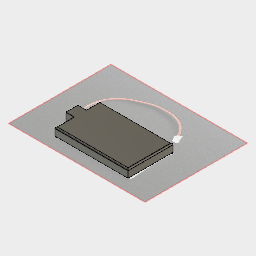
LiPo Battery (Autodesk Fusion 360 design; units mm, degrees)
Autodesk Fusion 360 part; units mm, degrees
sketch "Sketch1" plane through (0, 0, 0) normal (0, 0, 1) x (1, 0, 0) in component "LiPo_Battery"
  line L0 (33, 4) -> (-27, 4)
  line L1 (-27, -33) -> (33, -33)
  line L2 (33, -33) -> (33, 4)
  line L3 (-27, -8) -> (-33, -8)
  line L4 (-33, -8) -> (-33, -18)
  line L5 (-33, -18) -> (-27, -18)
  line L6 (-27, 4) -> (-27, -8)
  line L7 (-27, -18) -> (-27, -33)
  dimension "d4" = 60
  dimension "d5" = 37
  dimension "d6" = 6
  dimension "d7" = 10
  constraint horizontal L0
  constraint vertical L6
  constraint horizontal L1
  constraint vertical L2
  constraint horizontal L3
  constraint vertical L4
  constraint horizontal L5
  constraint collinear L6 L7
  measures "d5" distance of L0 L1
extrude "Extrude1" add sketch "Sketch1" along normal blind 7.5 in component "LiPo_Battery"
fillet "Fillet1" radius 1 10 edges at (3, -33, 7.5) (-27, -2, 7.5) (-27, -25.5, 7.5) (3, 4, 7.5) (33, -14.5, 7.5) (3, -33, 0) (33, -14.5, 0) (3, 4, 0) (-27, -25.5, 0) (-27, -2, 0) in component "LiPo_Battery"
sketch "Sketch2" plane through (0, 0, 7.5) normal (0, 0, 1) x (-1, 0, 0) in component "LiPo_Battery"
  line L0 (-32, -3) -> (26, -3)
  line L1 (26, 18) -> (26, 32)
  line L2 (26, 32) -> (-32, 32)
  line L3 (-32, 32) -> (-32, -3)
  line L4 (13.5433, 9.1078) -> (-24.3864, 9.1078)
  line L5 (-24.3864, 9.1078) -> (-24.3864, 5.1078)
  line L6 (-24.3864, 5.1078) -> (13.5433, 5.1078)
  line L7 (13.5433, 5.1078) -> (13.5433, 9.1078)
  line L8 (13.46, 17.9189) -> (-17.0674, 17.9189)
  line L9 (-17.0674, 17.9189) -> (-17.0674, 13.9189)
  line L10 (-17.0674, 13.9189) -> (13.46, 13.9189)
  line L11 (13.46, 13.9189) -> (13.46, 17.9189)
  line L12 (26, 8) -> (33, 8)
  line L13 (33, 8) -> (33, 18)
  line L14 (33, 18) -> (26, 18)
  line L15 (26, -3) -> (26, 8)
  constraint perpendicular L4 L5
  constraint parallel L4 L6
  constraint parallel L5 L7
  constraint perpendicular L8 L9
  constraint parallel L8 L10
  constraint parallel L9 L11
component "LiPo_Battery" placed x (1, 0, 0) y (0, 1, 0) z (0, 0, 1) at (0, 0, 0)
